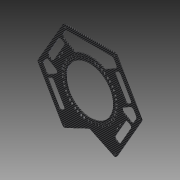
# Autodesk Inventor part: Bottom Plate
Saved by Autodesk Inventor 2015 (Build 190159000, 159)
## iProperties
Created: 2016-10-01
Part Number: Bottom Plate
Material: Generic
Document SubType Name: Modeling
Designer: James Yelland
Density: 1 g/cm^3
Appearance: Default
Author: James Yelland
Autodesk Inventor part; units mm, degrees
ref_plane "YZ Plane" through (0, 0, 0) normal (1, 0, 0) x (0, 1, 0)
ref_plane "XZ Plane" through (0, 0, 0) normal (0, 1, 0) x (-1, 0, 0)
ref_plane "XY Plane" through (0, 0, 0) normal (0, 0, 1) x (1, 0, 0)
sketch "Sketch1" plane through (0, 0, 0) normal (0, 1, 0) x (-1, 0, 0)
  line L0 (72.6878, -41.9663) -> (62.1878, -60.1529)
  line L1 (72.6878, -41.9663) -> (83.1878, -23.7798)
  line L2 (81.7237, -18.3157) -> (77.3936, -15.8157)
  line L3 (71.9295, -17.2797) -> (50.9295, -53.6529)
  line L4 (52.3936, -59.117) -> (56.7237, -61.617)
  arc A0 (56.7237, -61.617) -> (62.1878, -60.1529) centre (58.7237, -58.1529) ccw
  arc A1 (50.9295, -53.6529) -> (52.3936, -59.117) centre (54.3936, -55.6529) ccw
  arc A2 (77.3936, -15.8157) -> (71.9295, -17.2797) centre (75.3936, -19.2798) ccw
  arc A3 (83.1878, -23.7798) -> (81.7237, -18.3157) centre (79.7237, -21.7798) ccw
  line L5 (55.5994, -35.5644) -> (57.3314, -36.5644)
  line L6 (57.3314, -36.5644) -> (54.8314, -40.8945)
  line L7 (53.0994, -39.8945) -> (55.5994, -35.5644)
  line L8 (54.8314, -40.8945) -> (53.0994, -39.8945)
  line L9 (61.0994, -26.0381) -> (58.5994, -30.3683)
  line L10 (60.3314, -31.3683) -> (62.8314, -27.0381)
  line L11 (58.5994, -30.3683) -> (60.3314, -31.3683)
  line L12 (62.8314, -27.0381) -> (61.0994, -26.0381)
  line L13 (-72.6878, -41.9663) -> (-83.1878, -23.7798)
  line L14 (-72.6878, -41.9663) -> (-62.1878, -60.1529)
  line L15 (-56.7237, -61.617) -> (-52.3936, -59.117)
  line L16 (-50.9295, -53.6529) -> (-71.9294, -17.28)
  line L17 (-77.3936, -15.8157) -> (-81.7237, -18.3157)
  arc A4 (-81.7237, -18.3157) -> (-83.1878, -23.7798) centre (-79.7237, -21.7798) ccw
  arc A5 (-71.9294, -17.28) -> (-77.3936, -15.8157) centre (-75.3936, -19.2798) ccw
  arc A6 (-52.3936, -59.117) -> (-50.9295, -53.6529) centre (-54.3936, -55.6529) ccw
  arc A7 (-62.1878, -60.1529) -> (-56.7237, -61.617) centre (-58.7237, -58.1529) ccw
  line L18 (-58.5994, -30.3683) -> (-60.3314, -31.3683)
  line L19 (-61.0994, -26.0381) -> (-58.5994, -30.3683)
  line L20 (-62.8314, -27.0381) -> (-61.0994, -26.0381)
  line L21 (-60.3314, -31.3683) -> (-62.8314, -27.0381)
  line L22 (-54.8314, -40.8945) -> (-53.0994, -39.8945)
  line L23 (-53.0994, -39.8945) -> (-55.5994, -35.5644)
  line L24 (-55.5994, -35.5644) -> (-57.3314, -36.5644)
  line L25 (-57.3314, -36.5644) -> (-54.8314, -40.8945)
  line L26 (103.5566, -2.5) -> (54.8095, -86.9325)
  line L27 (-54.8095, -86.9325) -> (-103.5566, -2.5)
  line L28 (-103.5566, 2.5) -> (-53.9434, 88.4327)
  line L29 (-49.6132, 90.9327) -> (49.6132, 90.9327)
  line L30 (53.9434, 88.4327) -> (103.5566, 2.5)
  line L31 (2.1497, -66.9563) -> (48.3297, -88.9468)
  line L32 (-2.1497, -66.9563) -> (-48.3297, -88.9468)
  arc A8 (48.3297, -88.9468) -> (54.8095, -86.9325) centre (50.4794, -84.4325) ccw
  arc A9 (2.1497, -66.9563) -> (-2.1497, -66.9563) centre (0, -71.4706) ccw
  arc A10 (-54.8095, -86.9325) -> (-48.3297, -88.9468) centre (-50.4794, -84.4325) ccw
  arc A11 (-103.5566, 2.5) -> (-103.5566, -2.5) centre (-99.2265, 0) ccw
  arc A12 (-49.6132, 90.9327) -> (-53.9434, 88.4327) centre (-49.6132, 85.9327) ccw
  arc A13 (53.9434, 88.4327) -> (49.6132, 90.9327) centre (49.6132, 85.9327) ccw
  arc A14 (103.5566, -2.5) -> (103.5566, 2.5) centre (99.2265, 0) ccw
  circle A15 centre (49.6132, 85.9327) radius 1.6
  circle A16 centre (-49.6132, 85.9327) radius 1.6
  circle A17 centre (-99.2265, 0) radius 1.6
  circle A18 centre (99.2265, 0) radius 1.6
  arc A19 (48.9434, 79.7724) -> (44.6132, 82.2724) centre (44.6132, 77.2724) ccw
  arc A20 (-88.75, -10.8253) -> (-81.9199, -12.6554) centre (-84.4199, -8.3253) ccw
  arc A21 (-93.5566, 2.5) -> (-93.5566, -2.5) centre (-89.2265, 0) ccw
  arc A22 (81.9199, -12.6554) -> (88.75, -10.8253) centre (84.4199, -8.3253) ccw
  arc A23 (-44.6132, 82.2724) -> (-48.9434, 79.7724) centre (-44.6132, 77.2724) ccw
  arc A24 (93.5566, -2.5) -> (93.5566, 2.5) centre (89.2265, 0) ccw
  circle A25 centre (0, 0) radius 47.5
  circle A26 centre (50.4794, -84.4325) radius 1.6
  circle A27 centre (-50.4794, -84.4325) radius 1.6
  line L33 (0, -53.75) -> (-1.5, -53.75)
  line L34 (0, -53.75) -> (1.5, -53.75)
  line L35 (1.5, -53.75) -> (1.5, -56.75)
  line L36 (1.5, -56.75) -> (4.5, -56.75)
  line L37 (4.5, -56.75) -> (4.5, -50.75)
  line L38 (4.5, -50.75) -> (1.5, -50.75)
  line L39 (1.5, -50.75) -> (1.5, -53.75)
  line L40 (-1.5, -53.75) -> (-1.5, -56.75)
  line L41 (-1.5, -56.75) -> (-4.5, -56.75)
  line L42 (-1.5, -53.75) -> (-1.5, -53.75)
  line L43 (-1.5, -53.75) -> (-1.5, -50.75)
  line L44 (-1.5, -53.75) -> (1.5, -53.75) construction
  line L45 (-1.5, -50.75) -> (-4.5, -50.75)
  line L46 (-4.5, -56.75) -> (-4.5, -50.75)
  line L47 (15.3604, -51.5303) -> (16.1369, -54.4281)
  line L48 (16.1369, -54.4281) -> (19.0346, -53.6516)
  line L49 (19.0346, -53.6516) -> (17.4817, -47.856)
  line L50 (17.4817, -47.856) -> (14.584, -48.6325)
  line L51 (14.584, -48.6325) -> (15.3604, -51.5303)
  line L52 (12.4626, -52.3067) -> (13.2391, -55.2045)
  line L53 (13.2391, -55.2045) -> (10.3413, -55.981)
  line L54 (12.4626, -52.3067) -> (11.6862, -49.409)
  line L55 (11.6862, -49.409) -> (8.7884, -50.1854)
  line L56 (10.3413, -55.981) -> (8.7884, -50.1854)
  line L57 (28.174, -45.7989) -> (29.674, -48.3969)
  line L58 (29.674, -48.3969) -> (32.2721, -46.8969)
  line L59 (32.2721, -46.8969) -> (29.2721, -41.7008)
  line L60 (29.2721, -41.7008) -> (26.674, -43.2008)
  line L61 (26.674, -43.2008) -> (28.174, -45.7989)
  line L62 (25.576, -47.2989) -> (27.076, -49.8969)
  line L63 (27.076, -49.8969) -> (24.4779, -51.3969)
  line L64 (25.576, -47.2989) -> (24.076, -44.7008)
  line L65 (24.076, -44.7008) -> (21.4779, -46.2008)
  line L66 (24.4779, -51.3969) -> (21.4779, -46.2008)
  line L67 (39.0676, -36.9463) -> (41.189, -39.0676)
  line L68 (41.189, -39.0676) -> (43.3103, -36.9463)
  line L69 (43.3103, -36.9463) -> (39.0676, -32.7037)
  line L70 (39.0676, -32.7037) -> (36.9463, -34.825)
  line L71 (36.9463, -34.825) -> (39.0676, -36.9463)
  line L72 (36.9463, -39.0676) -> (39.0676, -41.189)
  line L73 (39.0676, -41.189) -> (36.9463, -43.3103)
  line L74 (36.9463, -39.0676) -> (34.825, -36.9463)
  line L75 (34.825, -36.9463) -> (32.7037, -39.0676)
  line L76 (36.9463, -43.3103) -> (32.7037, -39.0676)
  line L77 (47.2989, -25.576) -> (49.8969, -27.076)
  line L78 (49.8969, -27.076) -> (51.3969, -24.4779)
  line L79 (51.3969, -24.4779) -> (46.2008, -21.4779)
  line L80 (46.2008, -21.4779) -> (44.7008, -24.076)
  line L81 (44.7008, -24.076) -> (47.2989, -25.576)
  line L82 (45.7989, -28.174) -> (48.3969, -29.674)
  line L83 (48.3969, -29.674) -> (46.8969, -32.2721)
  line L84 (45.7989, -28.174) -> (43.2008, -26.674)
  line L85 (43.2008, -26.674) -> (41.7008, -29.2721)
  line L86 (46.8969, -32.2721) -> (41.7008, -29.2721)
  line L87 (52.3067, -12.4626) -> (55.2045, -13.2391)
  line L88 (55.2045, -13.2391) -> (55.981, -10.3413)
  line L89 (55.981, -10.3413) -> (50.1854, -8.7884)
  line L90 (50.1854, -8.7884) -> (49.409, -11.6862)
  line L91 (49.409, -11.6862) -> (52.3067, -12.4626)
  line L92 (51.5303, -15.3604) -> (54.4281, -16.1369)
  line L93 (54.4281, -16.1369) -> (53.6516, -19.0346)
  line L94 (51.5303, -15.3604) -> (48.6325, -14.584)
  line L95 (48.6325, -14.584) -> (47.856, -17.4817)
  line L96 (53.6516, -19.0346) -> (47.856, -17.4817)
  line L97 (53.75, 1.5) -> (56.75, 1.5)
  line L98 (56.75, 1.5) -> (56.75, 4.5)
  line L99 (56.75, 4.5) -> (50.75, 4.5)
  line L100 (50.75, 4.5) -> (50.75, 1.5)
  line L101 (50.75, 1.5) -> (53.75, 1.5)
  line L102 (53.75, -1.5) -> (56.75, -1.5)
  line L103 (56.75, -1.5) -> (56.75, -4.5)
  line L104 (53.75, -1.5) -> (50.75, -1.5)
  line L105 (50.75, -1.5) -> (50.75, -4.5)
  line L106 (56.75, -4.5) -> (50.75, -4.5)
  line L107 (51.5303, 15.3604) -> (54.4281, 16.1369)
  line L108 (54.4281, 16.1369) -> (53.6516, 19.0346)
  line L109 (53.6516, 19.0346) -> (47.856, 17.4817)
  line L110 (47.856, 17.4817) -> (48.6325, 14.584)
  line L111 (48.6325, 14.584) -> (51.5303, 15.3604)
  line L112 (52.3067, 12.4626) -> (55.2045, 13.2391)
  line L113 (55.2045, 13.2391) -> (55.981, 10.3413)
  line L114 (52.3067, 12.4626) -> (49.409, 11.6862)
  line L115 (49.409, 11.6862) -> (50.1854, 8.7884)
  line L116 (55.981, 10.3413) -> (50.1854, 8.7884)
  line L117 (45.7989, 28.174) -> (48.3969, 29.674)
  line L118 (48.3969, 29.674) -> (46.8969, 32.2721)
  line L119 (46.8969, 32.2721) -> (41.7008, 29.2721)
  line L120 (41.7008, 29.2721) -> (43.2008, 26.674)
  line L121 (43.2008, 26.674) -> (45.7989, 28.174)
  line L122 (47.2989, 25.576) -> (49.8969, 27.076)
  line L123 (49.8969, 27.076) -> (51.3969, 24.4779)
  line L124 (47.2989, 25.576) -> (44.7008, 24.076)
  line L125 (44.7008, 24.076) -> (46.2008, 21.4779)
  line L126 (51.3969, 24.4779) -> (46.2008, 21.4779)
  line L127 (36.9463, 39.0676) -> (39.0676, 41.189)
  line L128 (39.0676, 41.189) -> (36.9463, 43.3103)
  line L129 (36.9463, 43.3103) -> (32.7037, 39.0676)
  line L130 (32.7037, 39.0676) -> (34.825, 36.9463)
  line L131 (34.825, 36.9463) -> (36.9463, 39.0676)
  line L132 (39.0676, 36.9463) -> (41.189, 39.0676)
  line L133 (41.189, 39.0676) -> (43.3103, 36.9463)
  line L134 (39.0676, 36.9463) -> (36.9463, 34.825)
  line L135 (36.9463, 34.825) -> (39.0676, 32.7037)
  line L136 (43.3103, 36.9463) -> (39.0676, 32.7037)
  line L137 (25.576, 47.2989) -> (27.076, 49.8969)
  line L138 (27.076, 49.8969) -> (24.4779, 51.3969)
  line L139 (24.4779, 51.3969) -> (21.4779, 46.2008)
  line L140 (21.4779, 46.2008) -> (24.076, 44.7008)
  line L141 (24.076, 44.7008) -> (25.576, 47.2989)
  line L142 (28.174, 45.7989) -> (29.674, 48.3969)
  line L143 (29.674, 48.3969) -> (32.2721, 46.8969)
  line L144 (28.174, 45.7989) -> (26.674, 43.2008)
  line L145 (26.674, 43.2008) -> (29.2721, 41.7008)
  line L146 (32.2721, 46.8969) -> (29.2721, 41.7008)
  line L147 (12.4626, 52.3067) -> (13.2391, 55.2045)
  line L148 (13.2391, 55.2045) -> (10.3413, 55.981)
  line L149 (10.3413, 55.981) -> (8.7884, 50.1854)
  line L150 (8.7884, 50.1854) -> (11.6862, 49.409)
  line L151 (11.6862, 49.409) -> (12.4626, 52.3067)
  line L152 (15.3604, 51.5303) -> (16.1369, 54.4281)
  line L153 (16.1369, 54.4281) -> (19.0346, 53.6516)
  line L154 (15.3604, 51.5303) -> (14.584, 48.6325)
  line L155 (14.584, 48.6325) -> (17.4817, 47.856)
  line L156 (19.0346, 53.6516) -> (17.4817, 47.856)
  line L157 (-1.5, 53.75) -> (-1.5, 56.75)
  line L158 (-1.5, 56.75) -> (-4.5, 56.75)
  line L159 (-4.5, 56.75) -> (-4.5, 50.75)
  line L160 (-4.5, 50.75) -> (-1.5, 50.75)
  line L161 (-1.5, 50.75) -> (-1.5, 53.75)
  line L162 (1.5, 53.75) -> (1.5, 56.75)
  line L163 (1.5, 56.75) -> (4.5, 56.75)
  line L164 (1.5, 53.75) -> (1.5, 50.75)
  line L165 (1.5, 50.75) -> (4.5, 50.75)
  line L166 (4.5, 56.75) -> (4.5, 50.75)
  line L167 (-15.3604, 51.5303) -> (-16.1369, 54.4281)
  line L168 (-16.1369, 54.4281) -> (-19.0346, 53.6516)
  line L169 (-19.0346, 53.6516) -> (-17.4817, 47.856)
  line L170 (-17.4817, 47.856) -> (-14.584, 48.6325)
  line L171 (-14.584, 48.6325) -> (-15.3604, 51.5303)
  line L172 (-12.4626, 52.3067) -> (-13.2391, 55.2045)
  line L173 (-13.2391, 55.2045) -> (-10.3413, 55.981)
  line L174 (-12.4626, 52.3067) -> (-11.6862, 49.409)
  line L175 (-11.6862, 49.409) -> (-8.7884, 50.1854)
  line L176 (-10.3413, 55.981) -> (-8.7884, 50.1854)
  line L177 (-28.174, 45.7989) -> (-29.674, 48.3969)
  line L178 (-29.674, 48.3969) -> (-32.2721, 46.8969)
  line L179 (-32.2721, 46.8969) -> (-29.2721, 41.7008)
  line L180 (-29.2721, 41.7008) -> (-26.674, 43.2008)
  line L181 (-26.674, 43.2008) -> (-28.174, 45.7989)
  line L182 (-25.576, 47.2989) -> (-27.076, 49.8969)
  line L183 (-27.076, 49.8969) -> (-24.4779, 51.3969)
  line L184 (-25.576, 47.2989) -> (-24.076, 44.7008)
  line L185 (-24.076, 44.7008) -> (-21.4779, 46.2008)
  line L186 (-24.4779, 51.3969) -> (-21.4779, 46.2008)
  line L187 (-39.0676, 36.9463) -> (-41.189, 39.0676)
  line L188 (-41.189, 39.0676) -> (-43.3103, 36.9463)
  line L189 (-43.3103, 36.9463) -> (-39.0676, 32.7037)
  line L190 (-39.0676, 32.7037) -> (-36.9463, 34.825)
  line L191 (-36.9463, 34.825) -> (-39.0676, 36.9463)
  line L192 (-36.9463, 39.0676) -> (-39.0676, 41.189)
  line L193 (-39.0676, 41.189) -> (-36.9463, 43.3103)
  line L194 (-36.9463, 39.0676) -> (-34.825, 36.9463)
  line L195 (-34.825, 36.9463) -> (-32.7037, 39.0676)
  line L196 (-36.9463, 43.3103) -> (-32.7037, 39.0676)
  line L197 (-47.2989, 25.576) -> (-49.8969, 27.076)
  line L198 (-49.8969, 27.076) -> (-51.3969, 24.4779)
  line L199 (-51.3969, 24.4779) -> (-46.2008, 21.4779)
  line L200 (-46.2008, 21.4779) -> (-44.7008, 24.076)
  line L201 (-44.7008, 24.076) -> (-47.2989, 25.576)
  line L202 (-45.7989, 28.174) -> (-48.3969, 29.674)
  line L203 (-48.3969, 29.674) -> (-46.8969, 32.2721)
  line L204 (-45.7989, 28.174) -> (-43.2008, 26.674)
  line L205 (-43.2008, 26.674) -> (-41.7008, 29.2721)
  line L206 (-46.8969, 32.2721) -> (-41.7008, 29.2721)
  line L207 (-52.3067, 12.4626) -> (-55.2045, 13.2391)
  line L208 (-55.2045, 13.2391) -> (-55.981, 10.3413)
  line L209 (-55.981, 10.3413) -> (-50.1854, 8.7884)
  line L210 (-50.1854, 8.7884) -> (-49.409, 11.6862)
  line L211 (-49.409, 11.6862) -> (-52.3067, 12.4626)
  line L212 (-51.5303, 15.3604) -> (-54.4281, 16.1369)
  line L213 (-54.4281, 16.1369) -> (-53.6516, 19.0346)
  line L214 (-51.5303, 15.3604) -> (-48.6325, 14.584)
  line L215 (-48.6325, 14.584) -> (-47.856, 17.4817)
  line L216 (-53.6516, 19.0346) -> (-47.856, 17.4817)
  line L217 (-53.75, -1.5) -> (-56.75, -1.5)
  line L218 (-56.75, -1.5) -> (-56.75, -4.5)
  line L219 (-56.75, -4.5) -> (-50.75, -4.5)
  line L220 (-50.75, -4.5) -> (-50.75, -1.5)
  line L221 (-50.75, -1.5) -> (-53.75, -1.5)
  line L222 (-53.75, 1.5) -> (-56.75, 1.5)
  line L223 (-56.75, 1.5) -> (-56.75, 4.5)
  line L224 (-53.75, 1.5) -> (-50.75, 1.5)
  line L225 (-50.75, 1.5) -> (-50.75, 4.5)
  line L226 (-56.75, 4.5) -> (-50.75, 4.5)
  line L227 (-51.5303, -15.3604) -> (-54.4281, -16.1369)
  line L228 (-54.4281, -16.1369) -> (-53.6516, -19.0346)
  line L229 (-53.6516, -19.0346) -> (-47.856, -17.4817)
  line L230 (-47.856, -17.4817) -> (-48.6325, -14.584)
  line L231 (-48.6325, -14.584) -> (-51.5303, -15.3604)
  line L232 (-52.3067, -12.4626) -> (-55.2045, -13.2391)
  line L233 (-55.2045, -13.2391) -> (-55.981, -10.3413)
  line L234 (-52.3067, -12.4626) -> (-49.409, -11.6862)
  line L235 (-49.409, -11.6862) -> (-50.1854, -8.7884)
  line L236 (-55.981, -10.3413) -> (-50.1854, -8.7884)
  line L237 (-45.7989, -28.174) -> (-48.3969, -29.674)
  line L238 (-48.3969, -29.674) -> (-46.8969, -32.2721)
  line L239 (-46.8969, -32.2721) -> (-41.7008, -29.2721)
  line L240 (-41.7008, -29.2721) -> (-43.2008, -26.674)
  line L241 (-43.2008, -26.674) -> (-45.7989, -28.174)
  line L242 (-47.2989, -25.576) -> (-49.8969, -27.076)
  line L243 (-49.8969, -27.076) -> (-51.3969, -24.4779)
  line L244 (-47.2989, -25.576) -> (-44.7008, -24.076)
  line L245 (-44.7008, -24.076) -> (-46.2008, -21.4779)
  line L246 (-51.3969, -24.4779) -> (-46.2008, -21.4779)
  line L247 (-36.9463, -39.0676) -> (-39.0676, -41.189)
  line L248 (-39.0676, -41.189) -> (-36.9463, -43.3103)
  line L249 (-36.9463, -43.3103) -> (-32.7037, -39.0676)
  line L250 (-32.7037, -39.0676) -> (-34.825, -36.9463)
  line L251 (-34.825, -36.9463) -> (-36.9463, -39.0676)
  line L252 (-39.0676, -36.9463) -> (-41.189, -39.0676)
  line L253 (-41.189, -39.0676) -> (-43.3103, -36.9463)
  line L254 (-39.0676, -36.9463) -> (-36.9463, -34.825)
  line L255 (-36.9463, -34.825) -> (-39.0676, -32.7037)
  line L256 (-43.3103, -36.9463) -> (-39.0676, -32.7037)
  line L257 (-25.576, -47.2989) -> (-27.076, -49.8969)
  line L258 (-27.076, -49.8969) -> (-24.4779, -51.3969)
  line L259 (-24.4779, -51.3969) -> (-21.4779, -46.2008)
  line L260 (-21.4779, -46.2008) -> (-24.076, -44.7008)
  line L261 (-24.076, -44.7008) -> (-25.576, -47.2989)
  line L262 (-28.174, -45.7989) -> (-29.674, -48.3969)
  line L263 (-29.674, -48.3969) -> (-32.2721, -46.8969)
  line L264 (-28.174, -45.7989) -> (-26.674, -43.2008)
  line L265 (-26.674, -43.2008) -> (-29.2721, -41.7008)
  line L266 (-32.2721, -46.8969) -> (-29.2721, -41.7008)
  line L267 (-12.4626, -52.3067) -> (-13.2391, -55.2045)
  line L268 (-13.2391, -55.2045) -> (-10.3413, -55.981)
  line L269 (-10.3413, -55.981) -> (-8.7884, -50.1854)
  line L270 (-8.7884, -50.1854) -> (-11.6862, -49.409)
  line L271 (-11.6862, -49.409) -> (-12.4626, -52.3067)
  line L272 (-15.3604, -51.5303) -> (-16.1369, -54.4281)
  line L273 (-16.1369, -54.4281) -> (-19.0346, -53.6516)
  line L274 (-15.3604, -51.5303) -> (-14.584, -48.6325)
  line L275 (-14.584, -48.6325) -> (-17.4817, -47.856)
  line L276 (-19.0346, -53.6516) -> (-17.4817, -47.856)
  arc A28 (-83.1878, 23.7798) -> (-81.7237, 18.3157) centre (-79.7237, 21.7798) ccw
  line L277 (-81.7237, 18.3157) -> (-77.3936, 15.8157)
  arc A29 (-77.3936, 15.8157) -> (-71.9295, 17.2798) centre (-75.3936, 19.2798) ccw
  line L278 (-72.6878, 41.9663) -> (-83.1878, 23.7798)
  line L279 (-62.8314, 27.0381) -> (-61.0994, 26.0381)
  line L280 (-60.3314, 31.3683) -> (-62.8314, 27.0381)
  line L281 (-61.0994, 26.0381) -> (-58.5994, 30.3683)
  line L282 (-58.5994, 30.3683) -> (-60.3314, 31.3683)
  line L283 (-55.5994, 35.5644) -> (-57.3314, 36.5644)
  line L284 (-57.3314, 36.5644) -> (-54.8314, 40.8945)
  line L285 (-53.0994, 39.8945) -> (-55.5994, 35.5644)
  line L286 (-71.9295, 17.2798) -> (-50.9296, 53.6527)
  line L287 (-72.6878, 41.9663) -> (-62.1878, 60.1529)
  line L288 (-54.8314, 40.8945) -> (-53.0994, 39.8945)
  arc A30 (-56.7237, 61.617) -> (-62.1878, 60.1529) centre (-58.7237, 58.1529) ccw
  line L289 (-52.3936, 59.117) -> (-56.7237, 61.617)
  arc A31 (-50.9296, 53.6527) -> (-52.3936, 59.117) centre (-54.3936, 55.6529) ccw
  arc A32 (-53.75, 71.4471) -> (-51.9199, 64.617) centre (-49.4199, 68.9471) ccw
  arc A33 (-81.9199, 12.6554) -> (-88.75, 10.8253) centre (-84.4199, 8.3253) ccw
  arc A34 (-31.4758, 52.8136) -> (-28.5484, 52.773) centre (-29.9758, 55.4117) ccw
  arc A35 (62.1878, 60.1529) -> (56.7237, 61.6169) centre (58.7237, 58.1528) ccw
  line L290 (56.7237, 61.6169) -> (52.3936, 59.1169)
  arc A36 (52.3936, 59.1169) -> (50.9295, 53.6528) centre (54.3936, 55.6528) ccw
  line L291 (72.6878, 41.9663) -> (62.1878, 60.1529)
  line L292 (54.8314, 40.8945) -> (53.0994, 39.8945)
  line L293 (57.3314, 36.5644) -> (54.8314, 40.8945)
  line L294 (53.0994, 39.8945) -> (55.5994, 35.5644)
  line L295 (55.5994, 35.5644) -> (57.3314, 36.5644)
  line L296 (58.5994, 30.3683) -> (60.3314, 31.3683)
  line L297 (60.3314, 31.3683) -> (62.8314, 27.0381)
  line L298 (61.0994, 26.0381) -> (58.5994, 30.3683)
  line L299 (50.9295, 53.6528) -> (71.9294, 17.28)
  line L300 (72.6878, 41.9663) -> (83.1878, 23.7798)
  line L301 (62.8314, 27.0381) -> (61.0994, 26.0381)
  arc A37 (81.7237, 18.3157) -> (83.1878, 23.7798) centre (79.7237, 21.7798) ccw
  line L302 (77.3936, 15.8157) -> (81.7237, 18.3157)
  arc A38 (71.9294, 17.28) -> (77.3936, 15.8157) centre (75.3936, 19.2798) ccw
  arc A39 (88.75, 10.8253) -> (81.9199, 12.6554) centre (84.4199, 8.3253) ccw
  arc A40 (51.9199, 64.617) -> (53.75, 71.4471) centre (49.4199, 68.9471) ccw
  line L303 (51.9199, 64.617) -> (31.4758, 52.8136)
  arc A41 (28.5484, 52.773) -> (31.4758, 52.8136) centre (29.9758, 55.4117) ccw
  arc A42 (67.5, 4.3301) -> (67.5, -4.3301) centre (70, 0) ccw
  arc A43 (-67.5, -4.3301) -> (-67.5, 4.3301) centre (-70, 0) ccw
  line L304 (53.75, 71.4471) -> (48.9434, 79.7724)
  line L305 (44.6132, 82.2724) -> (-44.6132, 82.2724)
  line L306 (-48.9434, 79.7724) -> (-53.75, 71.4471)
  line L307 (-51.9199, 64.617) -> (-31.4758, 52.8136)
  arc A44 (28.5484, 52.773) -> (-28.5484, 52.773) centre (0, 0) ccw
  line L308 (-67.5, -4.3301) -> (-81.9199, -12.6554)
  line L309 (-88.75, -10.8253) -> (-93.5566, -2.5)
  line L310 (-93.5566, 2.5) -> (-88.75, 10.8253)
  line L311 (-81.9199, 12.6554) -> (-67.5, 4.3301)
  line L312 (81.9199, 12.6554) -> (67.5, 4.3301)
  line L313 (67.5, -4.3301) -> (81.9199, -12.6554)
  line L314 (88.75, -10.8253) -> (93.5566, -2.5)
  line L315 (93.5566, 2.5) -> (88.75, 10.8253)
  point P0 (60.1878, -63.617)
  point P1 (85.1878, -20.3157)
  point P2 (73.9295, -13.8157)
  point P3 (48.9295, -57.117)
  point P4 (-85.1878, -20.3157)
  point P5 (-60.1878, -63.617)
  point P6 (-48.9295, -57.117)
  point P7 (-73.9295, -13.8157)
  point P8 (105, 0)
  point P9 (52.5, -90.9327)
  point P10 (-105, 0)
  point P11 (-52.5, 90.9327)
  point P12 (52.5, 90.9327)
  point P13 (-86.25, -15.1554)
  point P14 (60, 0)
  point P15 (-60, 0)
  point P16 (-73.9295, 13.8157)
  point P17 (-85.1878, 20.3157)
  point P18 (-48.9295, 57.117)
  point P19 (-60.1878, 63.617)
  point P20 (-30, 51.9615)
  point P21 (-60, 0)
  point P22 (48.9295, 57.1169)
  point P23 (60.1878, 63.6169)
  point P24 (73.9295, 13.8157)
  point P25 (85.1878, 20.3157)
  point P26 (60, 0)
  point P27 (30, 51.9615)
  dimension "d11" = 360
  dimension "d30" = 360
  dimension "d32" = 5
  dimension "d82" = 5
  constraints: 632 end point, 76 point on circle, 66 point on line, 45 centre point, 7 coincident, 6 perpendicular, 1 equal radius, 1 horizontal, 1 parallel, 1 tangent
  measures "d32" radius of A23
  measures "d82" radius of A42
extrude "Extrusion1" add sketch "Sketch1" along normal blind 2
body "Solid1"
